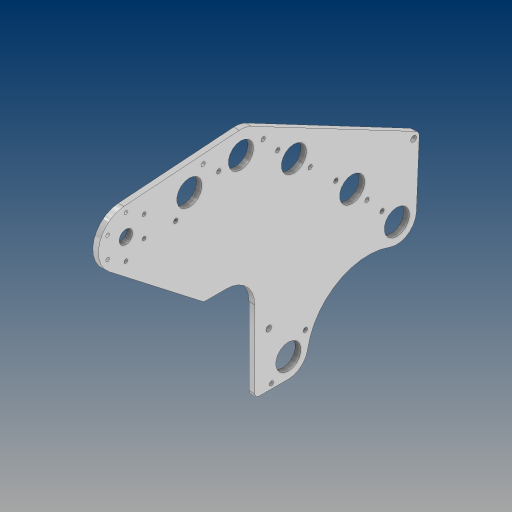
# Autodesk Inventor part: Intake Roller Plate
Saved by Autodesk Inventor 2024.3 (Build 283343000, 343)
## iProperties
Created: 2024-07-25
Part Number: Intake Roller Plate
Material: Aluminum 6061
Document SubType Name: Modeling
Designer: Kenji
Density: 2.7 g/cm^3
Appearance: Aluminum - Dark
Author: Kenji
Autodesk Inventor part; units mm, degrees
ref_plane "YZ Plane" through (0, 0, 0) normal (1, 0, 0) x (0, 1, 0)
ref_plane "XZ Plane" through (0, 0, 0) normal (0, 1, 0) x (-1, 0, 0)
ref_plane "XY Plane" through (0, 0, 0) normal (0, 0, 1) x (1, 0, 0)
sketch "Sketch1" plane through (0, 0, 0) normal (1, 0, 0) x (0, 1, 0)
  line L0 (127, 0) -> (127, -31.75) construction
  line L1 (95.25, -63.5) -> (31.75, -63.5) construction
  line L2 (0, -31.75) -> (0, 0) construction
  arc A0 (95.25, -63.5) -> (127, -31.75) centre (95.25, -31.75) ccw construction
  arc A1 (0, -31.75) -> (31.75, -63.5) centre (31.75, -31.75) ccw construction
  line L3 (0, 0) -> (0, 19.05) construction
  line L4 (0, 19.05) -> (-12.7, 19.05) construction
  line L5 (82.55, 19.05) -> (82.55, 292.1) construction
  circle A2 centre (82.55, 292.1) radius 25.4 construction
  circle A3 centre (82.55, 292.1) radius 31.75 construction
  circle A4 centre (231.775, 292.1) radius 25.4 construction
  circle A5 centre (231.775, 292.1) radius 31.75 construction
  line L6 (-12.7, 19.05) -> (82.55, 19.05) construction
  line L7 (127, 0) -> (0, 0) construction
  line L8 (-12.7, 19.05) -> (-12.7, -285.75) construction
  circle A6 centre (38.1, -175.1237) radius 50.8 construction
  circle A7 centre (96.0971, -224.5481) radius 25.4 construction
  circle A8 centre (96.0971, -224.5481) radius 14.2875
  circle A9 centre (153.6466, -173.8737) radius 25.4 construction
  circle A10 centre (153.6466, -173.8737) radius 14.2875
  circle A11 centre (249.9155, -47.8338) radius 22.225 construction
  circle A12 centre (249.9155, -47.8338) radius 25.4 construction
  circle A13 centre (249.9155, -47.8338) radius 14.2875
  line L9 (82.55, 19.05) -> (127, 19.05) construction
  line L10 (127, 19.05) -> (127, 0) construction
  circle A14 centre (153.6466, -173.8737) radius 22.225 construction
  circle A15 centre (96.0971, -224.5481) radius 22.225 construction
  circle A16 centre (25.4, -101.6) radius 25.4 construction
  circle A17 centre (25.4, -101.6) radius 23.8125 construction
  line L11 (25.4, -76.2) -> (25.4, -63.5) construction
  circle A18 centre (216.5234, -107.8815) radius 25.4 construction
  circle A19 centre (216.5234, -107.8815) radius 22.225 construction
  circle A20 centre (216.5234, -107.8815) radius 14.2875
  line L12 (0, -101.6) -> (-12.7, -101.6) construction
  circle A21 centre (64.1171, -79.375) radius 6.477 construction
  circle A22 centre (25.4, -101.6) radius 14.2875
  circle A23 centre (64.1171, -79.375) radius 3.2512
  circle A24 centre (84.9265, -149.1714) radius 50.8 construction
  circle A25 centre (144.1337, -98.2698) radius 50.8 construction
  circle A26 centre (105.5334, -118.9394) radius 50.8 construction
  circle A27 centre (168.1754, -243.5219) radius 3.2512
  circle A28 centre (242.5281, 10.5862) radius 14.2875
  circle A29 centre (242.5281, 10.5862) radius 22.225 construction
  line L13 (216.5234, -107.8815) -> (153.6466, -173.8737) construction
  line L14 (153.6466, -173.8737) -> (96.0971, -224.5481) construction
  line L15 (82.55, 19.05) -> (31.75, 19.05) construction
  line L16 (31.75, 19.05) -> (31.75, 292.1) construction
  line L17 (31.75, 292.1) -> (82.55, 292.1) construction
  circle A30 centre (242.5281, 10.5862) radius 7.62 construction
  line L18 (-12.7, -285.75) -> (571.5, -285.75) construction
  line L19 (571.5, -285.75) -> (571.5, 292.1) construction
  line L20 (31.75, 292.1) -> (571.5, 292.1) construction
  line L21 (127, 19.05) -> (571.5, 19.05) construction
  circle A31 centre (234.95, 82.55) radius 7.62
  circle A32 centre (234.95, 82.55) radius 23.8125 construction
  circle A33 centre (258.7625, 82.55) radius 2.0828
  circle A34 centre (234.95, 82.55) radius 27.94 construction
  circle A35 centre (234.95, 82.55) radius 31.115 construction
  circle A36 centre (246.8562, 103.1722) radius 2.0828
  circle A37 centre (223.0437, 103.1722) radius 2.0828
  circle A38 centre (211.1375, 82.55) radius 2.0828
  circle A39 centre (223.0437, 61.9278) radius 2.0828
  circle A40 centre (246.8562, 61.9278) radius 2.0828
  line L22 (-12.7, -63.5) -> (368.3, -63.5) construction
  circle A41 centre (168.1754, -243.5219) radius 6.4262 construction
  line L23 (368.3, -63.5) -> (368.3, -285.75) construction
  line L24 (7.043, -116.7676) -> (81.9407, -207.4149) construction
  circle A42 centre (64.1171, -79.375) radius 6.35 construction
  circle A43 centre (242.5281, 10.5862) radius 25.4 construction
  line L25 (242.5281, 10.5862) -> (249.9155, -47.8338) construction
  line L26 (82.55, 19.05) -> (141.3002, 19.05) construction
  line L27 (141.3002, 19.05) -> (141.3002, 209.55) construction
  line L28 (141.3002, 209.55) -> (82.55, 209.55) construction
  line L29 (82.55, 209.55) -> (82.55, 19.05) construction
  circle A44 centre (133.35, 12.7) radius 6.35 construction
  circle A45 centre (177.072, -42.6893) radius 50.8 construction
  circle A46 centre (177.8, -23.221) radius 50.8 construction
  circle A47 centre (25.4, -101.6) radius 22.225 construction
  line L30 (173.8597, -246.5194) -> (272.3831, -59.6815)
  line L31 (3.175, -101.6) -> (3.175, -68.2752)
  circle A48 centre (133.35, 12.7) radius 3.2512 construction
  arc A49 (272.3831, -59.6815) -> (275.252, -46.039) centre (249.9155, -47.8338) ccw
  arc A50 (168.1754, -249.9481) -> (173.8597, -246.5194) centre (168.1754, -243.5219) ccw
  arc A51 (3.175, -101.6) -> (21.6232, -123.5017) centre (25.4, -101.6) ccw
  arc A52 (7.9502, -63.5) -> (3.175, -68.2752) centre (7.9502, -68.2752) ccw
  arc A53 (265.9872, 84.7486) -> (210.3667, 101.6236) centre (234.95, 82.55) ccw
  line L32 (141.3002, 53.086) -> (157.9626, 53.086) construction
  line L33 (157.9626, 53.086) -> (157.9626, 86.106) construction
  line L34 (157.9626, 86.106) -> (141.3002, 86.106) construction
  line L35 (141.3002, 86.106) -> (141.3002, 53.086) construction
  line L36 (249.9155, -47.8338) -> (253.1021, -73.0332) construction
  line L37 (249.9155, -47.8338) -> (246.729, -22.6345) construction
  circle A54 centre (246.729, -22.6345) radius 2.4257
  circle A55 centre (253.1021, -73.0332) radius 2.4257
  line L38 (236.5065, 15.2558) -> (262.5999, -4.9792) construction
  line L39 (236.5065, 15.2558) -> (222.4562, 26.1515) construction
  circle A56 centre (262.5999, -4.9792) radius 2.4257
  circle A57 centre (222.4562, 26.1515) radius 2.4257
  circle A58 centre (262.5999, -4.9792) radius 5.6007 construction
  circle A59 centre (222.4562, 26.1515) radius 5.6007 construction
  circle A60 centre (246.729, -22.6345) radius 5.6007 construction
  circle A61 centre (253.1021, -73.0332) radius 5.6007 construction
  line L40 (216.5234, -107.8815) -> (234.0446, -89.4922) construction
  line L41 (216.5234, -107.8815) -> (199.0022, -126.2709) construction
  circle A62 centre (234.0446, -89.4922) radius 2.4257
  circle A63 centre (199.0022, -126.2709) radius 2.4257
  circle A64 centre (171.1678, -155.4844) radius 2.4257
  circle A65 centre (134.5835, -190.6594) radius 2.4257
  arc A66 (75.2683, -216.795) -> (95.1256, -246.7519) centre (96.0971, -224.5481) ccw
  circle A67 centre (8.7757, -82.396) radius 2.4257
  circle A68 centre (8.7757, -82.396) radius 5.6007 construction
  arc A69 (75.2683, -216.795) -> (21.6232, -123.5017) centre (9.7416, -192.4039) ccw
  line L42 (8.7757, -82.396) -> (42.0243, -120.804) construction
  circle A70 centre (42.0243, -120.804) radius 2.4257
  circle A71 centre (42.0243, -120.804) radius 5.6007 construction
  line L43 (7.9502, -63.5) -> (95.25, -63.5)
  arc A72 (95.25, -63.5) -> (127, -31.75) centre (95.25, -31.75) ccw
  line L44 (168.1754, -249.9481) -> (95.1256, -246.7519)
  circle A73 centre (115.1602, -207.7624) radius 2.4257
  line L45 (96.0971, -224.5481) -> (77.0341, -241.3339) construction
  line L46 (82.55, 133.35) -> (88.9, 133.35) construction
  line L47 (82.55, 184.15) -> (88.9, 184.15) construction
  line L48 (127, -31.75) -> (127, -7.4601)
  line L49 (265.9872, 84.7486) -> (275.252, -46.039)
  line L50 (128.0024, -4.5328) -> (210.3667, 101.6236)
  arc A74 (128.0024, -4.5328) -> (127, -7.4601) centre (131.7752, -7.4601) ccw
  line L51 (82.55, 44.45) -> (571.5, 44.45) construction
  line L52 (496.9444, 290.823) -> (300.0111, 214.4518) construction
  line L53 (503.4839, 289.6814) -> (556.5183, 239.3442) construction
  arc A75 (503.4839, 289.6814) -> (496.9444, 290.823) centre (499.2679, 284.8315) ccw construction
  arc A76 (551.8513, 203.7079) -> (556.5183, 239.3442) centre (541.2181, 223.2242) ccw construction
  arc A77 (551.8513, 203.7079) -> (531.1319, 98.1043) centre (585.3029, 142.3103) ccw construction
  arc A78 (530.6861, 69.4717) -> (531.1319, 98.1043) centre (513.9127, 84.0526) ccw construction
  circle A79 centre (513.9127, 84.0526) radius 22.225 construction
  line L54 (530.6861, 69.4717) -> (508.823, 44.3211) construction
  arc A80 (502.0863, 43.8501) -> (508.823, 44.3211) centre (505.2192, 47.454) ccw construction
  line L55 (502.0863, 43.8501) -> (436.2003, 101.1239) construction
  arc A81 (436.2003, 101.1239) -> (391.4084, 97.9917) centre (415.3705, 77.1619) ccw construction
  line L56 (391.4084, 97.9917) -> (375.4728, 79.6599) construction
  line L57 (372.7959, 78.1083) -> (240.9899, 52.0268) construction
  arc A82 (372.7959, 78.1083) -> (375.4728, 79.6599) centre (371.8689, 82.7927) ccw
  line L58 (210.0835, 101.2529) -> (288.8957, 206.0379) construction
  arc A83 (300.0111, 214.4518) -> (288.8957, 206.0379) centre (309.1949, 190.7702) ccw construction
  point P0 (-12.7, -175.1237)
  point P1 (179.0466, -173.8737)
  point P2 (104.775, 19.05)
  point P3 (174.6016, -243.5219)
  point P4 (127, -63.5)
  point P5 (3.175, -63.5)
  point P6 (96.0971, -249.9481)
  point P7 (127, -5.8248)
  point P8 (505.6902, 40.7173)
  point P9 (358.0806, 59.6525)
  point P10 (374.4, 78.4257)
  dimension "d58" = 101.6
  dimension "d267" = 15.24
  dimension "d284" = 47.625
  dimension "d2" = 31.75
  dimension "d3" = 19.05
  dimension "d4" = 12.7
  dimension "d7" = 273.05
  dimension "d8" = 50.8
  dimension "d9" = 6.35
  dimension "d10" = 50.8
  dimension "d11" = 6.35
  dimension "d12" = 149.225
  dimension "d14" = 127
  dimension "d16" = 304.8
  dimension "d175" = 31.75
  dimension "d180" = 50.8
  dimension "d181" = 1.5875
  dimension "d187" = 31.75
  dimension "d189" = 12.7
  dimension "d191" = 12.954
  dimension "d192" = 28.575
  dimension "d201" = 6.5024
  dimension "d207" = 101.6
  dimension "d208" = 101.6
  dimension "d210" = 130.175
  dimension "d214" = 15.875
  dimension "d218" = 6.5024
  dimension "d220" = 143.1895
  dimension "d236" = 50.8
  dimension "d237" = 44.45
  dimension "d271" = 584.2
  dimension "d283" = 15.24
  dimension "d285" = 4.1656
  dimension "d290" = 55.88
  dimension "d292" = 3.175
  dimension "d321" = 360
  dimension "d323" = 381
  dimension "d328" = 3.175
  dimension "d336" = 12.7
  dimension "d375" = 12.7
  dimension "d376" = 108.7971
  dimension "d377" = 76.6801
  dimension "d388" = 50.8
  dimension "d389" = 3.175
  dimension "d395" = 44.45
  dimension "d399" = 58.7502
  dimension "d400" = 190.5
  dimension "d404" = 12.7
  dimension "d405" = 101.6
  dimension "d406" = 101.6
  dimension "d407" = 58.42
  dimension "d409" = 3.175
  dimension "d410" = 6.5024
  dimension "d411" = 4.7752
  dimension "d427" = 16.6624
  dimension "d428" = 33.02
  dimension "d429" = 34.036
  dimension "d433" = 4.8514
  dimension "d434" = 4.8514
  dimension "d435" = 4.8514
  dimension "d436" = 4.8514
  dimension "d437" = 3.175
  dimension "d438" = 3.175
  dimension "d439" = 3.175
  dimension "d440" = 3.175
  dimension "d441" = 45
  dimension "d443" = 4.8514
  constraints: 119 end point, 80 centre point, 68 point on circle, 35 tangent, 32 point on line, 21 coincident, 18 equal radius, 16 perpendicular, 8 horizontal alignment, 8 parallel, 7 collinear, 7 concentric, 6 horizontal, 4 vertical, 2 midpoint, 2 vertical alignment, 72 other
  measures "d2" radius of A0
  measures "d3" distance of L2.end L3.end
  measures "d4" distance of L3.end L4.end
  measures "d7" distance of L5.start L5.end
  measures "d8" diameter of A2
  measures "d9" radial gap between concentric circles of A2 A3
  measures "d10" diameter of A4
  measures "d11" radial gap between concentric circles of A4 A5
  measures "d12" distance of L17.end A4.centre
  measures "d14" distance of L0.start L2.end
  measures "d16" distance of L4.end L8.end
  measures "d175" radius of A1
  measures "d180" diameter of A16
  measures "d187" distance of L0.start L0.end
  measures "d189" distance of L12.start L12.end
  measures "d191" diameter of A21
  measures "d192" diameter of A22
  measures "d201" diameter of A23
  measures "d207" diameter of A24
  measures "d208" diameter of A25
  measures "d210" distance of A21.centre A14.centre
  measures "d214" distance from line of L1 A21.centre
  measures "d218" diameter of A27
  measures "d220" distance of A0.centre A19.centre
  measures "d236" distance of L5.start L15.end
  measures "d237" distance of L4.end L15.end
  measures "d271" distance of L8.end L18.end
  measures "d283" diameter of A31
  measures "d285" diameter of A33
  measures "d290" diameter of A34
  measures "d292" radial gap between concentric circles of A34 A35
  measures "d323" distance of L22.start L22.end
  measures "d328" radial gap between concentric circles of A27 A41
  measures "d336" diameter of A42
  measures "d375" distance of L11.start L11.end
  measures "d376" distance from line of L8 A15.centre
  measures "d377" distance of L13.end L14.end
  measures "d388" diameter of A9
  measures "d389" radial gap between concentric circles of A15 A7
  measures "d395" diameter of A15
  measures "d399" distance of L28.end L27.end
  measures "d400" distance of L27.end L26.end
  measures "d404" diameter of A44
  measures "d405" diameter of A45
  measures "d406" diameter of A46
  measures "d407" vertical distance of L25.start L25.end
  measures "d409" radial gap between concentric circles of A16 A47
  measures "d410" diameter of A48
  measures "d411" radius of A52
  measures "d427" distance of L34.end L33.end
  measures "d428" distance between parallel lines of L32 L34
  measures "d429" distance from line of L26.end L32
  measures "d433" diameter of A54
  measures "d434" diameter of A55
  measures "d435" diameter of A56
  measures "d436" diameter of A57
  measures "d437" radial gap between concentric circles of A56 A58
  measures "d438" radial gap between concentric circles of A57 A59
  measures "d439" radial gap between concentric circles of A54 A60
  measures "d440" radial gap between concentric circles of A55 A61
  measures "d441" angle of L25 L38
  measures "d443" diameter of A62
extrude "Extrusion12" add sketch "Sketch1" along normal blind 6.35
body "Solid11"
